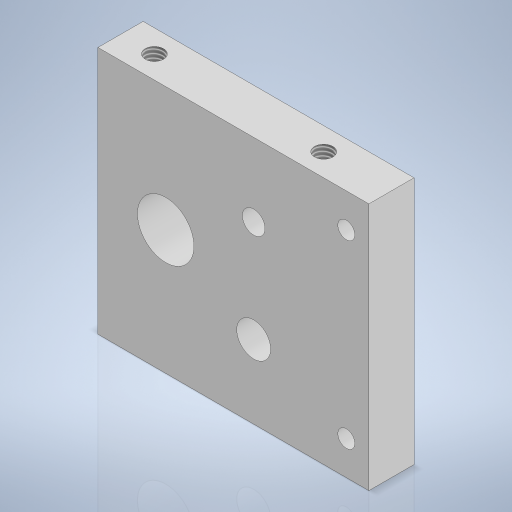
# Autodesk Inventor part: 1014
Saved by Autodesk Inventor 2024 (Build 280153000, 153)
## iProperties
Created: 2024-07-12
Part Number: 1014
Material: Generisch
Document SubType Name: Modeling
Designer: ffogue
Density: 1 g/cm^3
Appearance: Vorgabe
Author: ffogue
Autodesk Inventor part; units mm, degrees
note: some values were not read from the file. Chosen so that the rebuilt part matches the saved one: direction of "Bohrung2".
ref_plane "YZ Plane" through (0, 0, 0) normal (1, 0, 0) x (0, 1, 0)
ref_plane "XZ Plane" through (0, 0, 0) normal (0, 1, 0) x (-1, 0, 0)
sketch "Skizze1" plane through (0, 0, 0) normal (0, 1, 0) x (-1, 0, 0)
  line L0 (0, 0) -> (48, 0)
  line L1 (48, 0) -> (48, -44)
  line L2 (48, -44) -> (0, -44)
  line L3 (0, -44) -> (0, 0)
  dimension "d0" = 44
  dimension "d1" = 48
  constraints: 8 end point, 2 parallel, 1 horizontal, 1 perpendicular
  measures "d0" distance between parallel lines of L2 L0
  measures "d1" distance between parallel lines of L3 L1
extrude "Extrusion1" add sketch "Skizze1" along normal blind 8
sketch "Skizze2" plane through (0, 8, 0) normal (0, 1, 0) x (1, 0, 0)
  circle A0 centre (-36, 22) radius 5
  circle A1 centre (-20.4115, 13) radius 2
  circle A2 centre (-20.4115, 31) radius 3
  line L0 (0, 0) -> (0, 44) projected
  line L1 (0, 22) -> (-47.9314, 22) construction
  line L2 (-48, 44) -> (-48, 0) projected
  dimension "d4" = 9
  dimension "d5" = 12
  dimension "d6" = 10
  dimension "d7" = 18
  dimension "d8" = 4
  dimension "d9" = 6
  constraints: 3 centre point, 2 end point, 1 horizontal, 1 midpoint, 1 point on line, 1 symmetric about line, 1 vertical alignment
  measures "d4" distance from line of L1 A1.centre
  measures "d5" distance from line of L2 A0.centre
  measures "d6" diameter of A0
  measures "d7" distance of A1.centre A0.centre
  measures "d8" diameter of A1
  measures "d9" diameter of A2
extrude "Extrusion2" cut sketch "Skizze2" against normal up to surface (8 mm away)
sketch "Skizze3" plane through (-48, 0, -44) normal (-1, 0, 0) x (0, 0, 1)
  line L0 (44, 0) -> (44, 8) projected
  line L1 (0, 0) -> (44, 0) projected
  point P0 (22, 4)
  point P1 (44, 4)
  point P2 (22, 0)
  constraints: 2 midpoint, 1 horizontal alignment, 1 vertical alignment
hole "Bohrung1" at (-48, 4, -22) direction (1, 0, 0) diameter 3.242 depth 4 thread size "M4x0.7" class "6H" standard "ISO Metric profile"
sketch "Skizze4" plane through (0, 8, 0) normal (0, 1, 0) x (1, 0, 0)
  line L0 (0, 0) -> (0, 44) projected
  line L1 (-48, 0) -> (0, 0) projected
  point P0 (-4, 6)
  point P1 (-4, 38)
  dimension "d26" = 4
  dimension "d27" = 6
  dimension "d28" = 32
  constraints: 1 vertical alignment
  measures "d26" distance from line of L0 point (-4, 6)
  measures "d27" distance from line of L1 point (-4, 6)
  measures "d28" distance of point (-4, 38) point (-4, 6)
hole "Bohrung2" at (-4, 8, -6) at (-4, 8, -38) direction (0, -1, 0) diameter 3 depth 8
sketch "Skizze5" plane through (0, 0, -44) normal (0, 0, -1) x (-1, 0, 0)
  line L0 (48, 0) -> (48, 8) projected
  line L1 (0, 0) -> (0, 8) projected
  point P0 (12, 4)
  point P1 (42, 4)
  point P2 (48, 4)
  dimension "d36" = 30
  dimension "d37" = 12
  constraints: 2 horizontal alignment, 1 midpoint
  measures "d36" distance of point (12, 4) point (42, 4)
  measures "d37" distance from line of L1 point (12, 4)
hole "Bohrung3" at (-12, 4, -44) at (-42, 4, -44) direction (0, 0, 1) diameter 3.242 depth 10 thread size "M4x0.7" class "6H" standard "ISO Metric profile"
ref_plane "Arbeitsebene1" through (0, 0, -22) normal (0, 0, 1) x (1, 0, 0)
mirror "Spiegeln1" about plane through (0, 0, -22) normal (0, 0, 1) of "Bohrung3"
